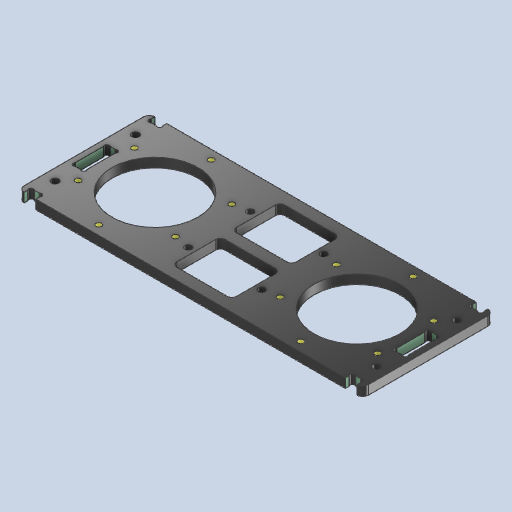
# Autodesk Inventor part: Trunk_waisit_frame
Saved by Autodesk Inventor 2022.3 (Build 263350000, 350)
## iProperties
Part Number: Trunk_waisit_frame
Material: アルミニウム 2014-T4
Document SubType Name: Modeling
Designer: Masato Kubotera
Density: 2.8 g/cm^3
Appearance: 光沢 - 黒
Mass: 54.9351 g
Surface Area: 142.462 cm^2
Volume: 19.6197 cm^3
Description: A2017 T4
Author: Masato Kubotera
Revision Number: Rev.2 Specifications for RoboCup 2023: Anodized aluminum staining process added.
Autodesk Inventor part; units mm, degrees
ref_plane "YZ Plane" through (0, 0, 0) normal (1, 0, 0) x (0, 1, 0)
ref_plane "XZ Plane" through (0, 0, 0) normal (0, 1, 0) x (-1, 0, 0)
ref_plane "XY Plane" through (0, 0, 0) normal (0, 0, 1) x (1, 0, 0)
derived "Outer_support_stand.ipt"
sketch "スケッチ1" plane through (0, 0, 0) normal (0, 0, 1) x (1, 0, 0)
  circle A0 centre (0, 0) radius 18.75 construction
  circle A1 centre (0, 0) radius 20.5 construction
  circle A2 centre (0, 0) radius 20.51 construction
  line L0 (0, 0) -> (0, 24.5) construction
  circle A3 centre (0, 24.5) radius 1.55 construction
  circle A4 centre (0, 24.5) radius 3 construction
  arc A5 (0, 28.5) -> (-3.7147, 25.9835) centre (0, 24.5) ccw construction
  arc A6 (-5.1639, 24.7674) -> (-18.8673, 16.8557) centre (0, 0) ccw construction
  arc A7 (-5.1639, 24.7674) -> (-3.7147, 25.9835) centre (-5.5721, 26.7253) ccw construction
  arc A8 (3.7147, 25.9835) -> (5.1639, 24.7674) centre (5.5721, 26.7253) ccw construction
  arc A9 (3.7147, 25.9835) -> (0, 28.5) centre (0, 24.5) ccw construction
  circle A10 centre (0, 24.5) radius 3.05 construction
  arc A11 (-24.0311, 7.9117) -> (-24.0311, -7.9117) centre (0, 0) ccw construction
  arc A12 (-24.0311, 7.9117) -> (-24.3598, 9.7747) centre (-25.9308, 8.5371) ccw construction
  arc A13 (-24.6817, 14.25) -> (-24.3598, 9.7747) centre (-21.2176, 12.25) ccw construction
  arc A14 (-20.645, 16.2088) -> (-24.6817, 14.25) centre (-21.2176, 12.25) ccw construction
  arc A15 (-20.645, 16.2088) -> (-18.8673, 16.8557) centre (-20.3588, 18.1882) ccw construction
  circle A16 centre (-21.2176, 12.25) radius 3.05 construction
  circle A17 centre (-21.2176, 12.25) radius 1.55 construction
  arc A18 (-18.8673, -16.8557) -> (-5.1639, -24.7674) centre (0, 0) ccw construction
  arc A19 (-18.8673, -16.8557) -> (-20.645, -16.2088) centre (-20.3588, -18.1882) ccw construction
  arc A20 (-24.6817, -14.25) -> (-20.645, -16.2088) centre (-21.2176, -12.25) ccw construction
  arc A21 (-24.3598, -9.7747) -> (-24.6817, -14.25) centre (-21.2176, -12.25) ccw construction
  arc A22 (-24.3598, -9.7747) -> (-24.0311, -7.9117) centre (-25.9308, -8.5371) ccw construction
  circle A23 centre (-21.2176, -12.25) radius 3.05 construction
  circle A24 centre (-21.2176, -12.25) radius 1.55 construction
  arc A25 (5.1639, -24.7674) -> (18.8673, -16.8557) centre (0, 0) ccw construction
  arc A26 (5.1639, -24.7674) -> (3.7147, -25.9835) centre (5.5721, -26.7253) ccw construction
  arc A27 (0, -28.5) -> (3.7147, -25.9835) centre (0, -24.5) ccw construction
  arc A28 (-3.7147, -25.9835) -> (0, -28.5) centre (0, -24.5) ccw construction
  arc A29 (-3.7147, -25.9835) -> (-5.1639, -24.7674) centre (-5.5721, -26.7253) ccw construction
  circle A30 centre (0, -24.5) radius 3.05 construction
  circle A31 centre (0, -24.5) radius 1.55 construction
  arc A32 (24.0311, -7.9117) -> (24.0311, 7.9117) centre (0, 0) ccw construction
  arc A33 (24.0311, -7.9117) -> (24.3598, -9.7747) centre (25.9308, -8.5371) ccw construction
  arc A34 (24.6817, -14.25) -> (24.3598, -9.7747) centre (21.2176, -12.25) ccw construction
  arc A35 (20.645, -16.2088) -> (24.6817, -14.25) centre (21.2176, -12.25) ccw construction
  arc A36 (20.645, -16.2088) -> (18.8673, -16.8557) centre (20.3588, -18.1882) ccw construction
  circle A37 centre (21.2176, -12.25) radius 3.05 construction
  circle A38 centre (21.2176, -12.25) radius 1.55 construction
  arc A39 (18.8673, 16.8557) -> (5.1639, 24.7674) centre (0, 0) ccw construction
  arc A40 (18.8673, 16.8557) -> (20.645, 16.2088) centre (20.3588, 18.1882) ccw construction
  arc A41 (24.6817, 14.25) -> (20.645, 16.2088) centre (21.2176, 12.25) ccw construction
  arc A42 (24.3598, 9.7747) -> (24.6817, 14.25) centre (21.2176, 12.25) ccw construction
  arc A43 (24.3598, 9.7747) -> (24.0311, 7.9117) centre (25.9308, 8.5371) ccw construction
  circle A44 centre (21.2176, 12.25) radius 3.05 construction
  circle A45 centre (21.2176, 12.25) radius 1.55 construction
sketch "スケッチ2" plane through (0, 0, 0) normal (0, 0, 1) x (1, 0, 0)
  line L0 (-119, 28.5) -> (31, 28.5)
  line L1 (31, 28.5) -> (31, -28.5)
  line L2 (31, -28.5) -> (-119, -28.5)
  line L3 (-119, -28.5) -> (-119, 28.5)
  line L4 (-119, 28.5) -> (31, -28.5) construction
  line L5 (31, 28.5) -> (-119, -28.5) construction
  line L6 (-119, 0) -> (31, 0) construction
  line L7 (-44, 28.5) -> (-44, -28.5) construction
  line L8 (23.5, 7.5) -> (28.5, 7.5) construction
  line L9 (28.5, 7.5) -> (28.5, -7.5) construction
  line L10 (28.5, -7.5) -> (23.5, -7.5) construction
  line L11 (23.5, -7.5) -> (23.5, 7.5) construction
  line L12 (23.5, 7.5) -> (28.5, -7.5) construction
  line L13 (28.5, 7.5) -> (23.5, -7.5) construction
  circle A0 centre (26, -17.5) radius 1.6
  line L14 (23.45, 7.55) -> (28.55, 7.55)
  line L15 (28.55, 7.55) -> (28.55, -7.55)
  line L16 (28.55, -7.55) -> (23.45, -7.55)
  line L17 (23.45, -7.55) -> (23.45, 7.55)
  line L18 (23.45, 7.55) -> (28.55, -7.55) construction
  line L19 (28.55, 7.55) -> (23.45, -7.55) construction
  arc A1 (24.9349, 7.55) -> (23.45, 6.0651) centre (24.1925, 6.8075) ccw
  line L20 (26, 7.5) -> (26, -7.5) construction
  line L21 (23.5, 0) -> (28.5, 0) construction
  arc A2 (28.55, 6.0651) -> (27.0651, 7.55) centre (27.8075, 6.8075) ccw
  arc A3 (23.45, -6.0651) -> (24.9349, -7.55) centre (24.1925, -6.8075) ccw
  arc A4 (27.0651, -7.55) -> (28.55, -6.0651) centre (27.8075, -6.8075) ccw
  circle A5 centre (0, 24.5) radius 1.55 construction
  circle A6 centre (-21.2176, 12.25) radius 1.55 construction
  circle A7 centre (-21.2176, -12.25) radius 1.55 construction
  circle A8 centre (0, -24.5) radius 1.55 construction
  circle A9 centre (21.2176, -12.25) radius 1.55 construction
  circle A10 centre (21.2176, 12.25) radius 1.55 construction
  circle A11 centre (0, 24.5) radius 1.25
  circle A12 centre (-21.2176, 12.25) radius 1.25
  circle A13 centre (-21.2176, -12.25) radius 1.25
  circle A14 centre (0, -24.5) radius 1.25
  circle A15 centre (21.2176, -12.25) radius 1.25
  circle A16 centre (21.2176, 12.25) radius 1.25
  circle A17 centre (26, 17.5) radius 1.6
  circle A18 centre (-114, -17.5) radius 1.6
  line L22 (-111.45, 7.55) -> (-116.55, 7.55)
  line L23 (-116.55, 7.55) -> (-116.55, -7.55)
  line L24 (-116.55, -7.55) -> (-111.45, -7.55)
  line L25 (-111.45, -7.55) -> (-111.45, 7.55)
  arc A19 (-111.45, 6.0651) -> (-112.9349, 7.55) centre (-112.1925, 6.8075) ccw
  arc A20 (-115.0651, 7.55) -> (-116.55, 6.0651) centre (-115.8075, 6.8075) ccw
  arc A21 (-112.9349, -7.55) -> (-111.45, -6.0651) centre (-112.1925, -6.8075) ccw
  arc A22 (-116.55, -6.0651) -> (-115.0651, -7.55) centre (-115.8075, -6.8075) ccw
  circle A23 centre (-88, 24.5) radius 1.25
  circle A24 centre (-66.7824, 12.25) radius 1.25
  circle A25 centre (-66.7824, -12.25) radius 1.25
  circle A26 centre (-88, -24.5) radius 1.25
  circle A27 centre (-109.2176, -12.25) radius 1.25
  circle A28 centre (-109.2176, 12.25) radius 1.25
  circle A29 centre (-114, 17.5) radius 1.6
  circle A30 centre (0, 0) radius 10.5 construction
  line L26 (0, 0) -> (0, 24.5) construction
  line L27 (-31, -16) -> (-31, 16) construction
  line L28 (-31, 16) -> (12, 16) construction
  line L29 (12, 16) -> (12, -16) construction
  line L30 (12, -16) -> (-31, -16) construction
  line L31 (-31, -16) -> (12, 16) construction
  line L32 (-31, 16) -> (12, -16) construction
  line L33 (-31, 0) -> (12, 0) construction
  line L34 (-31, -14.4) -> (-39.5, -14.4) construction
  line L35 (-39.5, -14.4) -> (-39.5, 14.4) construction
  line L36 (-31, 14.4) -> (-39.5, 14.4) construction
  line L37 (-1, -13.5) -> (-1, 13.5) construction
  line L38 (-1, 13.5) -> (-28, 13.5) construction
  line L39 (-28, 13.5) -> (-28, -13.5) construction
  line L40 (-28, -13.5) -> (-1, -13.5) construction
  line L41 (-1, -13.5) -> (-28, 13.5) construction
  line L42 (-1, 13.5) -> (-28, -13.5) construction
  circle A31 centre (-28, -13.5) radius 1.5
  circle A32 centre (-28, 13.5) radius 1.5
  circle A33 centre (-60, -13.5) radius 1.5
  circle A34 centre (-60, 13.5) radius 1.5
  circle A35 centre (0, 0) radius 18.75
  circle A36 centre (-28, -13.5) radius 2.75 construction
  circle A37 centre (-88, 0) radius 18.75
  line L43 (23.45, -28.5) -> (23.45, -26.9349)
  arc A38 (24.9349, -25.45) -> (23.45, -26.9349) centre (24.1925, -26.1925) ccw
  line L44 (24.9349, -25.45) -> (27.0651, -25.45)
  line L45 (28.55, -28.5) -> (28.55, -26.9349)
  arc A39 (28.55, -26.9349) -> (27.0651, -25.45) centre (27.8075, -26.1925) ccw
  line L46 (23.5, -25.5) -> (28.5, -25.5) construction
  line L47 (23.5, -25.5) -> (23.5, -28.5) construction
  line L48 (28.5, -25.5) -> (28.5, -28.5) construction
  line L49 (23.45, 28.5) -> (23.45, 26.9349)
  arc A40 (23.45, 26.9349) -> (24.9349, 25.45) centre (24.1925, 26.1925) ccw
  line L50 (24.9349, 25.45) -> (27.0651, 25.45)
  line L51 (28.55, 28.5) -> (28.55, 26.9349)
  arc A41 (27.0651, 25.45) -> (28.55, 26.9349) centre (27.8075, 26.1925) ccw
  line L52 (-111.45, -28.5) -> (-111.45, -26.9349)
  arc A42 (-111.45, -26.9349) -> (-112.9349, -25.45) centre (-112.1925, -26.1925) ccw
  line L53 (-112.9349, -25.45) -> (-115.0651, -25.45)
  line L54 (-116.55, -28.5) -> (-116.55, -26.9349)
  arc A43 (-115.0651, -25.45) -> (-116.55, -26.9349) centre (-115.8075, -26.1925) ccw
  line L55 (-111.45, 28.5) -> (-111.45, 26.9349)
  arc A44 (-112.9349, 25.45) -> (-111.45, 26.9349) centre (-112.1925, 26.1925) ccw
  line L56 (-112.9349, 25.45) -> (-115.0651, 25.45)
  line L57 (-116.55, 28.5) -> (-116.55, 26.9349)
  arc A45 (-116.55, 26.9349) -> (-115.0651, 25.45) centre (-115.8075, 26.1925) ccw
  circle A46 centre (26, -17.5) radius 3 construction
  line L58 (-55, -2.5) -> (-33, -2.5)
  line L59 (-31, -4.5) -> (-31, -21.5)
  line L60 (-33, -23.5) -> (-55, -23.5)
  line L61 (-57, -21.5) -> (-57, -4.5)
  line L62 (-57, -2.5) -> (-31, -23.5) construction
  line L63 (-31, -2.5) -> (-57, -23.5) construction
  arc A47 (-55, -2.5) -> (-57, -4.5) centre (-55, -4.5) ccw
  arc A48 (-57, -21.5) -> (-55, -23.5) centre (-55, -21.5) ccw
  arc A49 (-33, -23.5) -> (-31, -21.5) centre (-33, -21.5) ccw
  arc A50 (-31, -4.5) -> (-33, -2.5) centre (-33, -4.5) ccw
  line L64 (-55, 2.5) -> (-33, 2.5)
  line L65 (-31, 4.5) -> (-31, 21.5)
  line L66 (-33, 23.5) -> (-55, 23.5)
  line L67 (-57, 21.5) -> (-57, 4.5)
  arc A51 (-57, 4.5) -> (-55, 2.5) centre (-55, 4.5) ccw
  arc A52 (-55, 23.5) -> (-57, 21.5) centre (-55, 21.5) ccw
  arc A53 (-31, 21.5) -> (-33, 23.5) centre (-33, 21.5) ccw
  arc A54 (-33, 2.5) -> (-31, 4.5) centre (-33, 4.5) ccw
  circle A55 centre (0, 0) radius 18.75 construction
  point P0 (-44, 0)
  point P1 (0, 28.5)
  point P2 (0, -28.5)
  point P3 (26, 0)
  point P4 (26, 0)
  point P5 (27.0651, -7.55)
  point P6 (24.9349, -7.55)
  point P7 (23.45, -6.0651)
  point P8 (27.0651, 7.55)
  point P9 (28.55, 6.0651)
  point P10 (28.55, -6.0651)
  point P11 (-115.0651, 7.55)
  point P12 (-111.45, -6.0651)
  point P13 (-112.9349, -7.55)
  point P14 (-115.0651, -7.55)
  point P15 (-116.55, -6.0651)
  point P16 (-116.55, 6.0651)
  point P17 (-9.5, 0)
  point P18 (-14.5, 0)
  point P19 (26, -25.45)
  point P20 (23.45, -25.45)
  point P21 (-44, -13)
  dimension "d5" = 5
  dimension "d6" = 15
  dimension "d7" = 3.2
  dimension "d14" = 0.05
  dimension "d15" = 0.05
  dimension "d16" = 1.05
  dimension "d25" = 2.5
  dimension "d26" = 2.5
  dimension "d27" = 2.5
  dimension "d28" = 2.5
  dimension "d29" = 2.5
  dimension "d30" = 2.5
  dimension "d40" = 21
  dimension "d43" = 57
  dimension "d45" = 90
  dimension "d46" = 44
  dimension "d47" = 43
  dimension "d48" = 32
  dimension "d49" = 28.8
  dimension "d50" = 8.5
  dimension "d51" = 9.5
  dimension "d52" = 27
  dimension "d53" = 27
  dimension "d54" = 3
  dimension "d55" = 8.5
  dimension "d56" = 180
  dimension "d58" = 35
  dimension "d59" = 37.5
  dimension "d60" = 4.75
  dimension "d61" = 5.5
  dimension "d72" = 67.5
  dimension "d73" = 2.5
  dimension "d74" = 150
  dimension "d75" = 1.05
  dimension "d76" = 3
  dimension "d77" = 0.05
  dimension "d78" = 6
  dimension "d79" = 2
  dimension "d80" = 5
  dimension "d81" = 0
  dimension "d82" = 5
  dimension "d83" = 37.5
  constraints: 134 end point, 78 symmetric about line, 50 point on circle, 49 centre point, 27 point on line, 24 midpoint, 14 parallel, 12 perpendicular, 10 coincident, 8 tangent, 3 equal radius, 1 collinear, 1 horizontal, 31 other
  measures "d5" distance of L9.end L10.end
  measures "d6" distance of L8.end L9.end
  measures "d7" diameter of A0
  measures "d14" distance between parallel lines of L17 L11
  measures "d15" distance between parallel lines of L14 L8
  measures "d16" radius of A1
  measures "d25" diameter of A11
  measures "d26" diameter of A12
  measures "d27" diameter of A13
  measures "d28" diameter of A14
  measures "d29" diameter of A15
  measures "d30" diameter of A16
  measures "d40" diameter of A30
  measures "d43" distance of L0.end L1.end
  measures "d45" angle of L0 L26
  measures "d46" distance of A30.centre point (-44, 0)
  measures "d47" distance of L27.end L28.end
  measures "d48" distance of L28.end L29.end
  measures "d49" distance of L34.end L35.end
  measures "d50" distance of L34.start L34.end
  measures "d51" distance of A30.centre point (-9.5, 0)
  measures "d52" distance of L39.end L38.end
  measures "d53" distance of L38.end L37.end
  measures "d54" diameter of A31
  measures "d55" distance from line of point (-9.5, 0) L37
  measures "d56" angle of L26 L27
  measures "d58" distance of A0.centre A17.centre
  measures "d59" diameter of A35
  measures "d60" distance edge to line of A35 L11
  measures "d61" diameter of A36
  measures "d72" distance of point (-44, 0) L21.start
  measures "d73" distance of L6.end L21.end
  measures "d74" distance of L0.start L0.end
  measures "d75" radius of A38
  measures "d76" distance of L46.end L48.end
  measures "d77" distance between parallel lines of L46 L44
  measures "d78" diameter of A46
  measures "d79" radius of A47
  measures "d80" vertical distance of L7.end L60.start
  measures "d81" horizontal distance of L62.end L27.start
  measures "d82" distance of L58.start L64.start
  measures "d83" diameter of A55
extrude "押し出し1" add sketch "スケッチ2" along normal blind 4 contours L0 L57 A45 L56 A44 L55 L49 A40 L50 A41 L51 L1 L2 L45 A39 L44 A38 L43 L52 A42 L53 A43 L54 L3
fillet "フィレット1" radius 2.5 4 edges at (31, 28.5, 2) (31, -28.5, 2) (-119, -28.5, 2) (-119, 28.5, 2)
equation "\"d15\" = d14"
